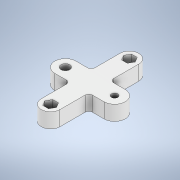
# Autodesk Inventor part: Acoplador
Saved by Autodesk Inventor 2020.3 (Build 243373000, 373)
## iProperties
Created: 2020-08-04
Part Number: Acoplador
Material: ABS Plastic
Document SubType Name: Modeling
Designer: juanp
Density: 1.06 g/cm^3
Appearance: Smooth - White
Author: juanp
Autodesk Inventor part; units mm, degrees
ref_plane "YZ Plane" through (0, 0, 0) normal (1, 0, 0) x (0, 1, 0)
ref_plane "XZ Plane" through (0, 0, 0) normal (0, 1, 0) x (-1, 0, 0)
ref_plane "XY Plane" through (0, 0, 0) normal (0, 0, 1) x (1, 0, 0)
sketch "Sketch1" plane through (0, 0, 0) normal (0, 1, 0) x (-1, 0, 0)
  circle A0 centre (0, 0) radius 2.55
  circle A1 centre (0, -63.56) radius 2.55
  line L0 (0, 0) -> (0, -63.56) construction
  line L1 (0, 0) -> (0, -63.56) construction
  line L2 (-7.55, 0) -> (-7.55, -20.23)
  line L3 (7.55, -63.56) -> (7.55, -43.33)
  arc A2 (7.55, 0) -> (-7.55, 0) centre (0, 0) ccw
  arc A3 (-7.55, -63.56) -> (7.55, -63.56) centre (0, -63.56) ccw
  line L4 (19.85, -31.78) -> (-19.85, -31.78) construction
  circle A4 centre (19.85, -31.78) radius 3.55
  circle A5 centre (-19.85, -31.78) radius 2.55
  line L5 (19.85, -31.78) -> (-19.85, -31.78) construction
  line L6 (19.85, -23.23) -> (10.55, -23.23)
  line L7 (-19.85, -40.33) -> (-10.55, -40.33)
  arc A6 (19.85, -40.33) -> (19.85, -23.23) centre (19.85, -31.78) ccw
  arc A7 (-19.85, -23.23) -> (-19.85, -40.33) centre (-19.85, -31.78) ccw
  line L8 (7.55, -40.33) -> (7.55, -23.23) construction
  line L9 (-7.55, -43.33) -> (-7.55, -63.56)
  line L10 (-7.55, -23.23) -> (-7.55, -40.33) construction
  line L11 (7.55, -20.23) -> (7.55, 0)
  line L12 (7.55, -23.23) -> (-7.55, -23.23) construction
  line L13 (-10.55, -23.23) -> (-19.85, -23.23)
  line L14 (10.55, -40.33) -> (19.85, -40.33)
  line L15 (-7.55, -40.33) -> (7.55, -40.33) construction
  arc A8 (7.55, -20.23) -> (10.55, -23.23) centre (10.55, -20.23) ccw
  arc A9 (-10.55, -23.23) -> (-7.55, -20.23) centre (-10.55, -20.23) ccw
  arc A10 (-7.55, -43.33) -> (-10.55, -40.33) centre (-10.55, -43.33) ccw
  arc A11 (10.55, -40.33) -> (7.55, -43.33) centre (10.55, -43.33) ccw
  point P0 (0, -31.78)
  point P1 (0, -31.78)
  point P2 (0, -31.78)
  dimension "d0" = 5.1
  dimension "d1" = 5.1
  dimension "d2" = 63.56
  dimension "d3" = 5
  dimension "d18" = 39.7
  dimension "d19" = 7.1
  dimension "d20" = 5.1
  dimension "d22" = 3
  dimension "d31" = 5
  constraints: 36 end point, 32 tangent, 18 parallel, 16 point on circle, 12 centre point, 9 point on line, 4 midpoint, 3 coincident, 3 equal radius, 2 collinear, 1 horizontal, 1 vertical
  measures "d0" diameter of A0
  measures "d1" diameter of A1
  measures "d2" distance of L0.start L0.end
  measures "d3" radial gap between concentric circles of A1 A3
  measures "d18" distance of L4.start L4.end
  measures "d19" diameter of A4
  measures "d20" diameter of A5
  measures "d22" radius of A8
  measures "d31" radial gap between concentric circles of A6 A4
extrude "Extrusion1" add sketch "Sketch1" along normal blind 12
sketch "Sketch5" plane through (0, 12, 0) normal (0, 1, 0) x (1, 0, 0)
  line L0 (2.3383, 4.05) -> (4.6765, 0)
  line L1 (4.6765, 0) -> (2.3383, -4.05)
  line L2 (2.3383, -4.05) -> (-2.3383, -4.05)
  line L3 (-2.3383, -4.05) -> (-4.6765, 0)
  line L4 (-4.6765, 0) -> (-2.3383, 4.05)
  line L5 (-2.3383, 4.05) -> (2.3383, 4.05)
  circle A0 centre (0, 63.56) radius 2.55 projected
  line L6 (-2.3383, 59.51) -> (-4.6765, 63.56)
  line L7 (-4.6765, 63.56) -> (-2.3383, 67.61)
  line L8 (-2.3383, 67.61) -> (2.3383, 67.61)
  line L9 (2.3383, 67.61) -> (4.6765, 63.56)
  line L10 (4.6765, 63.56) -> (2.3383, 59.51)
  line L11 (2.3383, 59.51) -> (-2.3383, 59.51)
  point P0 (0, 0)
  point P1 (0, 0)
  dimension "d23" = 8.1
  dimension "d24" = 8.1
  constraints: 24 end point, 2 coincident, 2 horizontal, 26 other
  measures "d23" distance between parallel lines of L5 L2
  measures "d24" distance between parallel lines of L8 L11
extrude "Extrusion4" cut sketch "Sketch5" against normal blind 8 contours L0 L1 L2 L3 L4 L5 | A0 | L6 L7 L8 L9 L10 L11
sketch "Sketch6" plane through (0, 0, 0) normal (0, -1, 0) x (1, 0, 0)
  circle A0 centre (-19.85, -31.78) radius 3.55 projected
  line L0 (-14.8, -28.8644) -> (-14.8, -34.6956)
  line L1 (-14.8, -34.6956) -> (-19.85, -37.6112)
  line L2 (-19.85, -37.6112) -> (-24.9, -34.6956)
  line L3 (-24.9, -34.6956) -> (-24.9, -28.8644)
  line L4 (-24.9, -28.8644) -> (-19.85, -25.9488)
  line L5 (-19.85, -25.9488) -> (-14.8, -28.8644)
  circle A1 centre (19.85, -31.78) radius 2.55 projected
  line L6 (15.8, -34.1183) -> (15.8, -29.4417)
  line L7 (15.8, -29.4417) -> (19.85, -27.1035)
  line L8 (19.85, -27.1035) -> (23.9, -29.4417)
  line L9 (23.9, -29.4417) -> (23.9, -34.1183)
  line L10 (23.9, -34.1183) -> (19.85, -36.4565)
  line L11 (19.85, -36.4565) -> (15.8, -34.1183)
  point P0 (0, 0)
  dimension "d27" = 10.1
  dimension "d28" = 8.1
  constraints: 24 end point, 2 coincident, 2 vertical, 26 other
  measures "d27" distance between parallel lines of L0 L3
  measures "d28" distance between parallel lines of L9 L6
extrude "Extrusion5" cut sketch "Sketch6" against normal blind 8
body "Solid1"
